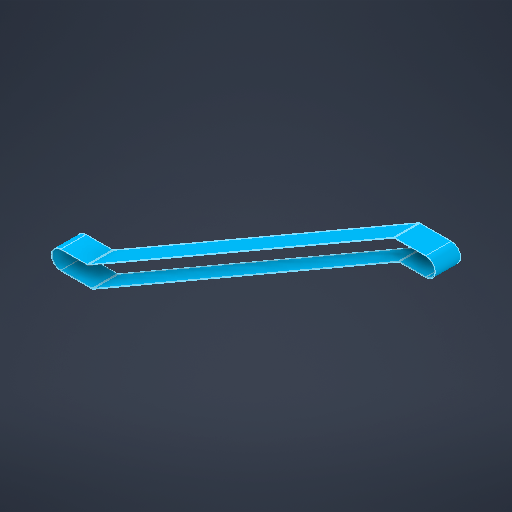
# Autodesk Inventor part: Assembly belt For lifting
Saved by Autodesk Inventor 2026.2 (Build 302298010, 298A)
## iProperties
Created: 2026-04-16
Part Number: Assembly belt For lifting
Material: Generic
Document SubType Name: Modeling
Designer: yassi
Density: 1 g/cm^3
Appearance: Sky Blue Medium
Author: yassi
Autodesk Inventor part; units mm, degrees
ref_plane "YZ Plane" through (0, 0, 0) normal (1, 0, 0) x (0, 1, 0)
ref_plane "XZ Plane" through (0, 0, 0) normal (0, 1, 0) x (-1, 0, 0)
ref_plane "XY Plane" through (0, 0, 0) normal (0, 0, 1) x (1, 0, 0)
sketch "Sketch1" plane through (0, 0, 0) normal (0, 0, 1) x (1, 0, 0)
  point P0 (0, 0)
sketch "Sketch2" plane through (0, 0, 0) normal (0, 0, 1) x (1, 0, 0)
  arc A0 (0, 15.5) -> (0, -15.5) centre (0, 0) ccw
  line L0 (0, 0) -> (50, 0) construction
  line L1 (50, 0) -> (569.6152, 300) construction
  line L2 (569.6152, 300) -> (619.6152, 300) construction
  arc A1 (619.6152, 284.5) -> (619.6152, 315.5) centre (619.6152, 300) ccw
  line L3 (619.6152, 315.5) -> (566.5338, 315.5)
  line L4 (564.5338, 314.9641) -> (46.775, 16.0359)
  line L5 (44.775, 15.5) -> (0, 15.5)
  line L6 (619.6152, 284.5) -> (574.8403, 284.5)
  line L7 (572.8403, 283.9641) -> (55.0814, -14.9641)
  line L8 (53.0814, -15.5) -> (0, -15.5)
  line L9 (46.641, 16.5359) -> (564.3999, 315.4641)
  line L10 (566.3999, 316) -> (619.6152, 316)
  arc A2 (619.6152, 284) -> (619.6152, 316) centre (619.6152, 300) ccw
  line L11 (619.6152, 284) -> (574.9742, 284)
  line L12 (572.9742, 283.4641) -> (55.2154, -15.4641)
  line L13 (53.2154, -16) -> (0, -16)
  arc A3 (0, 16) -> (0, -16) centre (0, 0) ccw
  line L14 (0, 16) -> (44.641, 16)
  line L15 (0, 15) -> (44.909, 15)
  line L16 (46.909, 15.5359) -> (564.6678, 314.4641)
  line L17 (566.6678, 315) -> (619.6152, 315)
  arc A4 (619.6152, 285) -> (619.6152, 315) centre (619.6152, 300) ccw
  line L18 (619.6152, 285) -> (574.7063, 285)
  line L19 (572.7063, 284.4641) -> (54.9474, -14.4641)
  line L20 (52.9474, -15) -> (0, -15)
  arc A5 (0, 15) -> (0, -15) centre (0, 0) ccw
  arc A6 (44.641, 16) -> (46.641, 16.5359) centre (44.641, 20) ccw
  arc A7 (44.775, 15.5) -> (46.775, 16.0359) centre (44.775, 19.5) ccw
  arc A8 (44.909, 15) -> (46.909, 15.5359) centre (44.909, 19) ccw
  arc A9 (52.9474, -15) -> (54.9474, -14.4641) centre (52.9474, -11) ccw
  arc A10 (53.0814, -15.5) -> (55.0814, -14.9641) centre (53.0814, -11.5) ccw
  arc A11 (53.2154, -16) -> (55.2154, -15.4641) centre (53.2154, -12) ccw
  arc A12 (574.7063, 285) -> (572.7063, 284.4641) centre (574.7063, 281) ccw
  arc A13 (574.8403, 284.5) -> (572.8403, 283.9641) centre (574.8403, 280.5) ccw
  arc A14 (574.9742, 284) -> (572.9742, 283.4641) centre (574.9742, 280) ccw
  arc A15 (566.3999, 316) -> (564.3999, 315.4641) centre (566.3999, 312) ccw
  arc A16 (566.5338, 315.5) -> (564.5338, 314.9641) centre (566.5338, 311.5) ccw
  arc A17 (566.6678, 315) -> (564.6678, 314.4641) centre (566.6678, 311) ccw
  dimension "d0" = 31
  dimension "d1" = 50
  dimension "d2" = 600
  dimension "d3" = 150
  dimension "d4" = 50
  dimension "d5" = 31
  dimension "d6" = 4
  dimension "d7" = 4
  dimension "d8" = 4
  dimension "d9" = 4
  dimension "d10" = 4
  dimension "d11" = 4
  dimension "d12" = 4
  dimension "d13" = 4
  dimension "d14" = 4
  dimension "d15" = 4
  constraints: 42 end point, 36 point on circle, 24 tangent, 18 centre point, 2 coincident, 2 equal radius, 1 horizontal, 1 parallel
  measures "d0" diameter of A0
  measures "d1" distance of L0.start L0.end
  measures "d2" distance of L0.end L1.end
  measures "d3" angle of L1 L0
  measures "d4" distance of L1.end L2.end
  measures "d5" diameter of A1
  measures "d6" radius of A6
  measures "d7" radius of A7
  measures "d8" radius of A8
  measures "d9" radius of A9
  measures "d10" radius of A12
  measures "d11" radius of A13
  measures "d12" radius of A14
  measures "d13" radius of A15
  measures "d14" radius of A16
  measures "d15" radius of A17
extrude "Extrusion1" add sketch "Sketch2" along normal blind 43 contours L5 A7 L4 A16 L3 A1 L6 A13 L7 A10 L8 A0 | L9 A15 L10 A2 L11 A14 L12 A11 L13 A3 L14 A6
body "Solid1"
